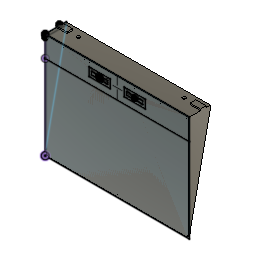
Key_Holder (Autodesk Fusion 360 design; units mm, degrees)
Autodesk Fusion 360 part; units mm, degrees
sketch "Sketch1" plane through (0, 0, 0) normal (0, 1, 0) x (1, 0, 0)
  line L0 (0, 0) -> (205, 0)
  line L1 (205, 0) -> (205, -120)
  line L2 (205, -120) -> (0, -120)
  line L3 (0, -120) -> (0, 0)
  line L4 (0, -120) -> (0, -150)
  line L5 (0, -150) -> (205, -150)
  line L6 (205, -150) -> (205, -120)
  circle A0 centre (127.5, -135) radius 3.25
  line L7 (112.5, -141) -> (142.5, -141)
  line L8 (142.5, -141) -> (142.5, -129)
  line L9 (142.5, -129) -> (112.5, -129)
  line L10 (112.5, -129) -> (112.5, -141)
  line L11 (112.5, -141) -> (142.5, -129) construction
  line L12 (142.5, -141) -> (112.5, -129) construction
  line L13 (116, -137.25) -> (139, -137.25)
  line L14 (139, -137.25) -> (139, -132.75)
  line L15 (139, -132.75) -> (116, -132.75)
  line L16 (116, -132.75) -> (116, -137.25)
  line L17 (116, -137.25) -> (139, -132.75) construction
  line L18 (139, -137.25) -> (116, -132.75) construction
  line L19 (102.5, -120) -> (102.5, -150) construction
  line L20 (62.5, -141) -> (92.5, -141)
  line L21 (92.5, -141) -> (92.5, -129)
  line L22 (92.5, -129) -> (62.5, -129)
  line L23 (62.5, -129) -> (62.5, -141)
  line L24 (62.5, -141) -> (92.5, -129) construction
  line L25 (92.5, -141) -> (62.5, -129) construction
  line L26 (66, -137.25) -> (89, -137.25)
  line L27 (89, -137.25) -> (89, -132.75)
  line L28 (89, -132.75) -> (66, -132.75)
  line L29 (66, -132.75) -> (66, -137.25)
  line L30 (66, -137.25) -> (89, -132.75) construction
  line L31 (89, -137.25) -> (66, -132.75) construction
  circle A1 centre (77.5, -135) radius 5
  line L32 (127.5, -135) -> (77.5, -135) construction
  point P0 (127.5, -135)
  point P1 (127.5, -135)
  point P2 (77.5, -135)
  point P3 (77.5, -135)
  dimension "d1" = 205
  dimension "d2" = 120
  dimension "d3" = 30
  dimension "d20" = 6.5
  dimension "d21" = 4.5
  dimension "d22" = 23
  dimension "d23" = 12
  dimension "d24" = 30
  dimension "d25" = 10
  dimension "d26" = 50
  constraint horizontal L0
  constraint vertical L1
  constraint horizontal L2
  constraint vertical L3
  constraint coincident L0.start L3.end
  constraint perpendicular L2 L4
  constraint perpendicular L3 L5
  constraint vertical L6
  constraint horizontal L7
  constraint perpendicular L7 L8
  constraint parallel L7 L9
  constraint parallel L8 L10
  constraint coincident L11 P1
  constraint coincident L12 P1
  constraint coincident P1 P0
  constraint horizontal L13
  constraint perpendicular L13 L14
  constraint parallel L13 L15
  constraint parallel L14 L16
  constraint coincident L17 P1
  constraint coincident L18 P1
  constraint midpoint L2 L19.start
  constraint midpoint L5 L19.end
  constraint horizontal L20
  constraint perpendicular L20 L21
  constraint parallel L20 L22
  constraint parallel L21 L23
  constraint coincident L24 P3
  constraint coincident L25 P3
  constraint horizontal L26
  constraint perpendicular L26 L27
  constraint parallel L26 L28
  constraint parallel L27 L29
  constraint coincident L30 P3
  constraint coincident L31 P3
  constraint coincident P3 P2
  constraint equal L10 L21
  constraint equal L7 L20
  constraint equal L13 L26
  constraint midpoint L19 L32
  constraint horizontal L32
  constraint equal L14 L27
  measures "d1" distance of L0.start L0.end
  measures "d2" distance of L0.end L1.end
  measures "d3" distance of L1.end L5.end
  measures "d20" diameter of A0
  measures "d21" distance of L13.start L15.end
  measures "d22" distance of L14.end L15.end
  measures "d23" distance of L7.end L8.end
  measures "d24" distance of L8.end L9.end
  measures "d25" diameter of A1
  measures "d26" distance of P1 P3
sketch "Sketch2" plane through (0, 0, 0) normal (1, 0, 0) x (0, 1, 0)
  line L0 (0, 120) -> (0, 0)
  line L1 (0, 120) -> (0, 150)
  line L2 (0, 0) -> (1, 0)
  line L3 (1, 0) -> (1, 8.3211)
  line L4 (0, 150) -> (30, 150)
  line L5 (30, 150) -> (30, 146)
  line L6 (30, 146) -> (1, 8.3211)
  line L7 (30, 146) -> (0, 146)
  line L8 (24, 150) -> (24, 152)
  line L9 (24, 152) -> (16, 152)
  line L10 (16, 152) -> (16, 150)
  line L11 (1, 8.3211) -> (1, 146)
  point P0 (20, 152)
  dimension "d4" = 1
  dimension "d5" = 4
  dimension "d6" = 30
  dimension "d7" = 2
  dimension "d8" = 8
  dimension "d9" = 20
  constraint coincident L0.end L2.start
  constraint perpendicular L0 L2
  constraint perpendicular L2 L3
  constraint coincident L1.end L4.start
  constraint perpendicular L1 L4
  constraint perpendicular L4 L5
  constraint coincident L1 L7.end
  constraint perpendicular L1 L7
  constraint coincident L4 L8.start
  constraint perpendicular L4 L8
  constraint perpendicular L8 L9
  constraint coincident L4 L10.end
  constraint perpendicular L4 L10
  constraint midpoint L9 P0
  constraint coincident L7 L11.end
  constraint perpendicular L7 L11
  measures "d4" distance of L2.end L0.end
  measures "d5" distance of L4 L7
  measures "d6" distance of L1.end L4.end
  measures "d7" distance of L8.start L8.end
  measures "d8" distance of L8.end L9.end
  measures "d9" horizontal distance of L1.end P0
extrude "Extrude1" add sketch "Sketch2" along normal up to surface (205 mm away) contours L0 L1 L2 L3 L7 L11 | L1 L4 L5 L7
extrude "Extrude2" add sketch "Sketch2" along normal blind 5 contours L6 L7 L11
fillet "Fillet1" chord length 10 1 edges at (2.5, 1, 8.3211)
pattern_linear "R-Pattern1" count 5 spacing 50 along (1, 0, 0) of "Extrude2", "Fillet1"
extrude "Extrude3" add sketch "Sketch1" along normal blind 13 contours A0 L13 L15 | A0 L13 L14 L15 | A0 L15 | A0 L13 | A0 L13 L15 L16 | L7 L8 L9 L10 | L20 L21 L22 L23 | L26 L28 L29 A1 | L26 L28 A1 | L26 A1 | L26 L27 L28 A1 | L28 A1
extrude "Extrude4" cut sketch "Sketch1" against normal blind 2 from surface at 13 contours A0 L13 L15 | A0 L13 L14 L15 | A0 L13 L15 L16 | L26 L28 L29 A1 | L26 L28 A1 | L26 L27 L28 A1
extrude "Extrude5" cut sketch "Sketch1" along normal through all contours A0 L13 L15 | A0 L15 | A0 L13 | L26 L28 A1 | L26 A1 | L28 A1
sketch "Sketch3" plane through (0, 0, 146) normal (0, 0, -1) x (1, 0, 0)
  line L0 (200, -30) -> (200, -1)
  line L1 (200, -1) -> (155, -1)
  line L2 (155, -1) -> (155, -30)
  line L3 (155, -30) -> (200, -30)
  line L4 (50, -30) -> (50, -1)
  line L5 (50, -1) -> (5, -1)
  line L6 (5, -1) -> (5, -30)
  line L7 (5, -30) -> (50, -30)
  line L8 (177.5, -30) -> (177.5, -1)
  line L9 (27.5, -30) -> (27.5, -1)
  point P0 (177.5, -20)
  point P1 (27.5, -20)
  dimension "d33" = 20
  constraint midpoint L3 L8.start
  constraint midpoint L1 L8.end
  constraint midpoint L7 L9.start
  constraint midpoint L5 L9.end
  constraint coincident L9 P1
  constraint coincident L8 P0
  constraint horizontal P0 P1
  measures "d33" vertical distance of P1 origin
hole "Hole1" at (177.5, 20, 146) at (27.5, 20, 146) direction (0, 0, 1) diameter 4.5 end through all countersink diameter 8 countersink angle 90
fillet "Fillet2" chord length 10 2 edges at (0, 0.5, 0) (205, 0.5, 0)
ref_plane "WorkPlane1" through (102.5, 15, 78.5355) normal (1, 0, 0) x (0, 0, -1)
extrude "Extrude6" add sketch "Sketch2" along normal blind 15 contours L4 L8 L9 L10
mirror "Mirror1" about plane through (102.5, 15, 78.5355) normal (1, 0, 0) of "Extrude6"
chamfer "Chamfer1" distance 0.6 angle 45 1 faces at (94.5375, 0, 43.3751)
